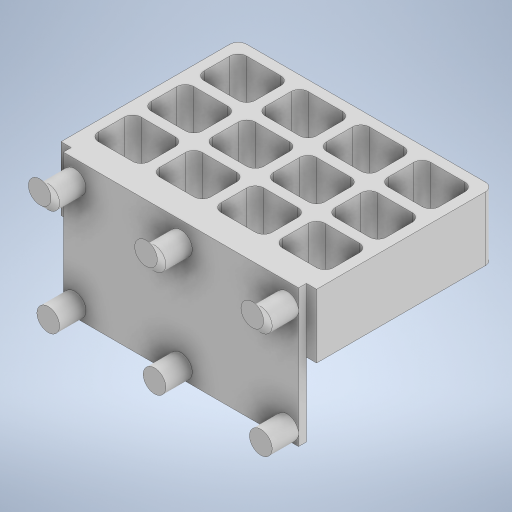
# Autodesk Inventor part: InvPegstr
Saved by Autodesk Inventor 2024 (Build 280153000, 153)
## iProperties
Created: 2024-12-11
Part Number: InvPegstr
Material: Типовые
Document SubType Name: Modeling
Designer: Admin
Density: 1 g/cm^3
Appearance: По умолчанию
Author: Admin
Autodesk Inventor part; units mm, degrees
ref_plane "YZ Plane" through (0, 0, 0) normal (1, 0, 0) x (0, 1, 0)
ref_plane "XZ Plane" through (0, 0, 0) normal (0, 1, 0) x (-1, 0, 0)
sketch "Эскиз1" plane through (0, 0, 0) normal (0, 0, 1) x (1, 0, 0)
  line L0 (-27.6, 16.125) -> (27.6, 16.125)
  line L1 (27.6, 16.125) -> (27.6, -16.125)
  line L2 (27.6, -16.125) -> (-27.6, -16.125)
  line L3 (-27.6, -16.125) -> (-27.6, 16.125)
  line L4 (-27.6, 16.125) -> (27.6, -16.125) construction
  line L5 (27.6, 16.125) -> (-27.6, -16.125) construction
  point P0 (0, 0)
  dimension "d2" = 55.2
  dimension "d3" = 32.25
  constraints: 12 end point, 2 midpoint, 2 parallel, 1 horizontal, 1 perpendicular
  measures "d2" distance of L0.start L0.end
  measures "d3" distance of L2.end L0.start
extrude "Выдавливание1" add sketch "Эскиз1" along normal blind 1.85
sketch "Эскиз2" plane through (0, 0, 1.85) normal (0, 0, 1) x (1, 0, 0)
  line L0 (-27.6, 16.125) -> (-27.6, -16.125) construction
  circle A0 centre (-24.95, 11.475) radius 2.65
  line L1 (0, 0) -> (0, 16.125) construction
  line L2 (27.6, 16.125) -> (-27.6, 16.125) construction
  line L3 (0, 0) -> (-27.6, 0) construction
  dimension "d4" = 5.3
  dimension "d51" = 2
  constraints: 4 end point, 2 midpoint, 1 centre point, 1 tangent
  measures "d4" diameter of A0
  measures "d51" distance edge to line of A0 L2
extrude "Выдавливание2" add sketch "Эскиз2" along normal blind 6.2
pattern_linear "Прямоуг.массив1" count 3 spacing 24.95 along (1, 0, 0) count 2 spacing 24.95 along (0, -1, 0) of "Выдавливание2"
sketch "Эскиз3" plane through (-27.6, 16.125, 0) normal (0, -1, 0) x (1, 0, 0)
  line L0 (57.6, -41.6) -> (-2.4, -41.6)
  line L1 (-2.4, -41.6) -> (-2.4, 0)
  line L2 (-2.4, 0) -> (57.6, 0)
  line L3 (57.6, 0) -> (57.6, -41.6)
  line L4 (0, 0) -> (55.2, 0) projected
  point P0 (27.6, 0)
  point P1 (27.6, 0)
  point P2 (27.6, 0)
  dimension "d46" = 60
  dimension "d47" = 41.6
  constraints: 8 end point, 3 midpoint, 2 coincident, 2 parallel, 1 horizontal, 1 perpendicular
  measures "d46" distance of L0.start L0.end
  measures "d47" distance of L0.end L1.end
extrude "Выдавливание3" add sketch "Эскиз3" along normal blind 15
sketch "Эскиз4" plane through (-27.6, 16.125, 1.85) normal (0, 1, 0) x (1, 0, 0)
  line L0 (55.2, 31.05) -> (43.2, 31.05)
  line L1 (43.2, 31.05) -> (43.2, 41.05)
  line L2 (43.2, 41.05) -> (55.2, 41.05)
  line L3 (55.2, 41.05) -> (55.2, 31.05)
  line L4 (-2.4, 43.45) -> (57.6, 43.45) projected
  line L5 (57.6, 43.45) -> (57.6, 1.85) projected
  point P0 (27.375, 1.85)
  point P1 (57.6, 1.85)
  dimension "d27" = 12
  dimension "d31" = 10
  dimension "d55" = 2.4
  dimension "d56" = 2.4
  constraints: 8 end point, 2 perpendicular, 1 other
  measures "d27" distance of L1.end L2.end
  measures "d31" distance of L0.end L1.end
  measures "d55" distance between parallel lines of L4 L2
extrude "Выдавливание4" cut sketch "Эскиз4" against normal blind 13
fillet "Сопряжение1" radius 2 4 edges at (15.6, 9.625, -29.2) (15.6, 9.625, -39.2) (27.6, 9.625, -29.2) (27.6, 9.625, -39.2)
pattern_linear "Прямоуг.массив2" count 4 spacing 14.4 along (-1, 0, 0) count 3 spacing 12.4 along (0, 0, 1) of "Выдавливание4", "Сопряжение1"
fillet "Сопряжение2" radius 2 2 edges at (30, 8.625, -41.6) (-30, 8.625, -41.6)
ref_plane "РабПлоскость1" through (-24.95, 11.475, 10.05) normal (0, 0, 1) x (1, 0, 0)
sketch "Эскиз7" plane through (-24.95, 11.475, 10.05) normal (0, 0, 1) x (1, 0, 0)
  circle A0 centre (0, 0) radius 2.65 construction
  circle A1 centre (0, 2) radius 2.65
  point P0 (24.95, -11.475)
  dimension "d60" = 5.3
  dimension "d61" = 2
  constraints: 1 centre point, 1 vertical alignment
  measures "d60" diameter of A1
  measures "d61" distance of A0.centre A1.centre
loft "Лофт1" add profiles "Эскиз7" section 1 edges at (-27.6, 11.475, 8.05)
pattern_linear "Прямоуг.массив3" count 3 spacing 24.95 along (1, 0, 0) of "Лофт1"
equation "\"d2\" = iTotalWidth"
equation "\"d3\" = iTotalHeight"
equation "\"iTotalWidth\" = 55.2"
equation "\"iTotalHeight\" = 32.25"
equation "\"iTotalHolderYSize\" = 41.6"
